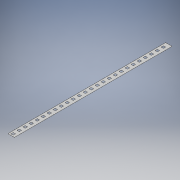
# Autodesk Inventor part: 1sqr metal plate
Saved by Autodesk Inventor 2018 (Build 220112000, 112)
## iProperties
Created: 2018-11-08
Part Number: 1sqr metal plate
Material: Generic
Document SubType Name: Modeling
Designer: USER
Density: 1 g/cm^3
Appearance: Default
Author: USER
Autodesk Inventor part; units mm, degrees
ref_plane "YZ Plane" through (0, 0, 0) normal (1, 0, 0) x (0, 1, 0)
ref_plane "XZ Plane" through (0, 0, 0) normal (0, 1, 0) x (-1, 0, 0)
ref_plane "XY Plane" through (0, 0, 0) normal (0, 0, 1) x (1, 0, 0)
sketch "Sketch1" plane through (0, 0, 0) normal (0, 1, 0) x (-1, 0, 0)
  line L0 (0, 0) -> (13, 0)
  line L1 (13, 0) -> (13, -315)
  line L2 (13, -315) -> (0, -315)
  line L3 (0, -315) -> (0, 0)
  dimension "d0" = 13
  dimension "d1" = 315
  constraints: 8 end point, 2 parallel, 1 horizontal, 1 perpendicular
  measures "d0" distance of L1.end L2.end
  measures "d1" distance of L0.end L1.end
extrude "Extrusion1" add sketch "Sketch1" along normal blind 0.1
sketch "Sketch2" plane through (0, 0.1, 0) normal (0, 1, 0) x (1, 0, 0)
  line L0 (-9.69, 2.7126) -> (-5.118, 2.7126)
  line L1 (-5.118, 2.7126) -> (-5.118, 7.2846)
  line L2 (-5.118, 7.2846) -> (-9.69, 7.2846)
  line L3 (-9.69, 7.2846) -> (-9.69, 2.7126)
  line L4 (-9.69, 14.7126) -> (-5.118, 14.7126)
  line L5 (-5.118, 14.7126) -> (-5.118, 19.2846)
  line L6 (-5.118, 19.2846) -> (-9.69, 19.2846)
  line L7 (-9.69, 19.2846) -> (-9.69, 14.7126)
  line L8 (-9.69, 26.7126) -> (-5.118, 26.7126)
  line L9 (-5.118, 26.7126) -> (-5.118, 31.2846)
  line L10 (-5.118, 31.2846) -> (-9.69, 31.2846)
  line L11 (-9.69, 31.2846) -> (-9.69, 26.7126)
  line L12 (-9.69, 38.7126) -> (-5.118, 38.7126)
  line L13 (-5.118, 38.7126) -> (-5.118, 43.2846)
  line L14 (-5.118, 43.2846) -> (-9.69, 43.2846)
  line L15 (-9.69, 43.2846) -> (-9.69, 38.7126)
  line L16 (-9.69, 50.7126) -> (-5.118, 50.7126)
  line L17 (-5.118, 50.7126) -> (-5.118, 55.2846)
  line L18 (-5.118, 55.2846) -> (-9.69, 55.2846)
  line L19 (-9.69, 55.2846) -> (-9.69, 50.7126)
  line L20 (-9.69, 62.7126) -> (-5.118, 62.7126)
  line L21 (-5.118, 62.7126) -> (-5.118, 67.2846)
  line L22 (-5.118, 67.2846) -> (-9.69, 67.2846)
  line L23 (-9.69, 67.2846) -> (-9.69, 62.7126)
  line L24 (-9.69, 74.7126) -> (-5.118, 74.7126)
  line L25 (-5.118, 74.7126) -> (-5.118, 79.2846)
  line L26 (-5.118, 79.2846) -> (-9.69, 79.2846)
  line L27 (-9.69, 79.2846) -> (-9.69, 74.7126)
  line L28 (-9.69, 86.7126) -> (-5.118, 86.7126)
  line L29 (-5.118, 86.7126) -> (-5.118, 91.2846)
  line L30 (-5.118, 91.2846) -> (-9.69, 91.2846)
  line L31 (-9.69, 91.2846) -> (-9.69, 86.7126)
  line L32 (-9.69, 98.7126) -> (-5.118, 98.7126)
  line L33 (-5.118, 98.7126) -> (-5.118, 103.2846)
  line L34 (-5.118, 103.2846) -> (-9.69, 103.2846)
  line L35 (-9.69, 103.2846) -> (-9.69, 98.7126)
  line L36 (-9.69, 110.7126) -> (-5.118, 110.7126)
  line L37 (-5.118, 110.7126) -> (-5.118, 115.2846)
  line L38 (-5.118, 115.2846) -> (-9.69, 115.2846)
  line L39 (-9.69, 115.2846) -> (-9.69, 110.7126)
  line L40 (-9.69, 122.7126) -> (-5.118, 122.7126)
  line L41 (-5.118, 122.7126) -> (-5.118, 127.2846)
  line L42 (-5.118, 127.2846) -> (-9.69, 127.2846)
  line L43 (-9.69, 127.2846) -> (-9.69, 122.7126)
  line L44 (-9.69, 134.7126) -> (-5.118, 134.7126)
  line L45 (-5.118, 134.7126) -> (-5.118, 139.2846)
  line L46 (-5.118, 139.2846) -> (-9.69, 139.2846)
  line L47 (-9.69, 139.2846) -> (-9.69, 134.7126)
  line L48 (-9.69, 146.7126) -> (-5.118, 146.7126)
  line L49 (-5.118, 146.7126) -> (-5.118, 151.2846)
  line L50 (-5.118, 151.2846) -> (-9.69, 151.2846)
  line L51 (-9.69, 151.2846) -> (-9.69, 146.7126)
  line L52 (-9.69, 158.7126) -> (-5.118, 158.7126)
  line L53 (-5.118, 158.7126) -> (-5.118, 163.2846)
  line L54 (-5.118, 163.2846) -> (-9.69, 163.2846)
  line L55 (-9.69, 163.2846) -> (-9.69, 158.7126)
  line L56 (-9.69, 170.7126) -> (-5.118, 170.7126)
  line L57 (-5.118, 170.7126) -> (-5.118, 175.2846)
  line L58 (-5.118, 175.2846) -> (-9.69, 175.2846)
  line L59 (-9.69, 175.2846) -> (-9.69, 170.7126)
  line L60 (-9.69, 182.7126) -> (-5.118, 182.7126)
  line L61 (-5.118, 182.7126) -> (-5.118, 187.2846)
  line L62 (-5.118, 187.2846) -> (-9.69, 187.2846)
  line L63 (-9.69, 187.2846) -> (-9.69, 182.7126)
  line L64 (-9.69, 194.7126) -> (-5.118, 194.7126)
  line L65 (-5.118, 194.7126) -> (-5.118, 199.2846)
  line L66 (-5.118, 199.2846) -> (-9.69, 199.2846)
  line L67 (-9.69, 199.2846) -> (-9.69, 194.7126)
  line L68 (-9.69, 206.7126) -> (-5.118, 206.7126)
  line L69 (-5.118, 206.7126) -> (-5.118, 211.2846)
  line L70 (-5.118, 211.2846) -> (-9.69, 211.2846)
  line L71 (-9.69, 211.2846) -> (-9.69, 206.7126)
  line L72 (-9.69, 218.7126) -> (-5.118, 218.7126)
  line L73 (-5.118, 218.7126) -> (-5.118, 223.2846)
  line L74 (-5.118, 223.2846) -> (-9.69, 223.2846)
  line L75 (-9.69, 223.2846) -> (-9.69, 218.7126)
  line L76 (-9.69, 230.7126) -> (-5.118, 230.7126)
  line L77 (-5.118, 230.7126) -> (-5.118, 235.2846)
  line L78 (-5.118, 235.2846) -> (-9.69, 235.2846)
  line L79 (-9.69, 235.2846) -> (-9.69, 230.7126)
  line L80 (-9.69, 242.7126) -> (-5.118, 242.7126)
  line L81 (-5.118, 242.7126) -> (-5.118, 247.2846)
  line L82 (-5.118, 247.2846) -> (-9.69, 247.2846)
  line L83 (-9.69, 247.2846) -> (-9.69, 242.7126)
  line L84 (-9.69, 254.7126) -> (-5.118, 254.7126)
  line L85 (-5.118, 254.7126) -> (-5.118, 259.2846)
  line L86 (-5.118, 259.2846) -> (-9.69, 259.2846)
  line L87 (-9.69, 259.2846) -> (-9.69, 254.7126)
  line L88 (-9.69, 266.7126) -> (-5.118, 266.7126)
  line L89 (-5.118, 266.7126) -> (-5.118, 271.2846)
  line L90 (-5.118, 271.2846) -> (-9.69, 271.2846)
  line L91 (-9.69, 271.2846) -> (-9.69, 266.7126)
  line L92 (-9.69, 278.7126) -> (-5.118, 278.7126)
  line L93 (-5.118, 278.7126) -> (-5.118, 283.2846)
  line L94 (-5.118, 283.2846) -> (-9.69, 283.2846)
  line L95 (-9.69, 283.2846) -> (-9.69, 278.7126)
  line L96 (-9.69, 290.7126) -> (-5.118, 290.7126)
  line L97 (-5.118, 290.7126) -> (-5.118, 295.2846)
  line L98 (-5.118, 295.2846) -> (-9.69, 295.2846)
  line L99 (-9.69, 295.2846) -> (-9.69, 290.7126)
  line L100 (-9.69, 302.7126) -> (-5.118, 302.7126)
  line L101 (-5.118, 302.7126) -> (-5.118, 307.2846)
  line L102 (-5.118, 307.2846) -> (-9.69, 307.2846)
  line L103 (-9.69, 307.2846) -> (-9.69, 302.7126)
  point P0 (0, 0)
  dimension "d4" = 4.572
  dimension "d5" = 4.572
  dimension "d8" = 12
  constraints: 208 end point, 2 parallel, 1 collinear, 1 horizontal, 1 perpendicular, 1 vertical, 199 other
  measures "d4" distance of L2.end L1.end
  measures "d5" distance of L1.end L0.end
  measures "d8" distance of L0.start L4.start
extrude "Extrusion2" cut sketch "Sketch2" against normal blind 0.1
body "Solid1"
